Autodesk Fusion 360 part; units mm, degrees
note: some values were not read from the file. Chosen so that the rebuilt part matches the saved one: which bodies a step acts on.
(part 2 of 4)
extrude "Extrude3''''''''''''''" cut sketch "Wedge_Pocket" against normal blind 42.5 from surface at -35 bodies 12 in component "Front_Wedge_L"
sketch "Wedge_HoldDown_Tap" plane through (0, 0, 0) normal (0, 0, 1) x (1, 0, 0) in component "Front_Wedge_L"
  circle A0 centre (-73, 80) radius 1.25
  circle A1 centre (-50, 50) radius 1.25
extrude "Extrude4''''''''''" cut sketch "Wedge_HoldDown_Tap" along normal blind 10 from surface at 5 bodies 12 in component "Front_Wedge_L"
sketch "Wedge_Pocket (2)" plane through (0, 0, 0) normal (1, 0, 0) x (0, 0, -1) in component "Front_Wedge_R"
  line L0 (-7.5, 42.5) -> (-7.5, 85.4279)
  line L1 (-7.5, 85.4279) -> (-74.4675, 42.5)
  line L2 (-74.4675, 42.5) -> (-7.5, 42.5)
extrude "Extrude3'''''''''''''''" cut sketch "Wedge_Pocket (2)" along normal blind 42.5 from surface at 35 bodies 13 in component "Front_Wedge_R"
sketch "Wedge_HoldDown_Tap (2)" plane through (0, 0, 0) normal (0, 0, 1) x (1, 0, 0) in component "Front_Wedge_R"
  circle A0 centre (50, 50) radius 1.25
  circle A1 centre (73, 80) radius 1.25
extrude "Extrude4'''''''''''" cut sketch "Wedge_HoldDown_Tap (2)" along normal blind 10 from surface at 5 bodies 13 in component "Front_Wedge_R"
sketch "Weapon_Pulley_Sketch" plane through (0, 0, 0) normal (1, 0, 0) x (0, 0, -1) in component "Weapon_Pulley"
  circle A0 centre (-38.5, 75) radius 10
extrude "Extrude1'''''''''''''''''''''''''''''" add sketch "Weapon_Pulley_Sketch" along normal blind 6 from surface at 16 separate body makes body 35 in component "Weapon_Pulley"
sketch "Motor_Pulley_Sketch" plane through (0, 0, 0) normal (1, 0, 0) x (0, 0, -1) in component "Motor_Pulley"
  circle A0 centre (-38.5, 25.75) radius 10
extrude "Extrude1''''''''''''''''''''''''''''''" add sketch "Motor_Pulley_Sketch" along normal blind 6 from surface at 16 separate body makes body 36 in component "Motor_Pulley"
sketch "Tension_Slot_-11_16" plane through (0, 0, 0) normal (0, 0, 1) x (1, 0, 0) in component "Base_Plate_Al"
  line L0 (-12.7, 13) -> (-9.3, 13)
  line L1 (-9.3, 13) -> (-9.3, 19)
  line L2 (-9.3, 19) -> (-12.7, 19)
  line L3 (-12.7, 19) -> (-12.7, 13)
extrude "Extrude15'" cut sketch "Tension_Slot_-11_16" along normal blind 6 from surface at 1 bodies 1 in component "Base_Plate_Al"
sketch "Tension_Slot_11_16" plane through (0, 0, 0) normal (0, 0, 1) x (1, 0, 0) in component "Base_Plate_Al"
  line L0 (9.3, 13) -> (12.7, 13)
  line L1 (12.7, 13) -> (12.7, 19)
  line L2 (12.7, 19) -> (9.3, 19)
  line L3 (9.3, 19) -> (9.3, 13)
extrude "Extrude16" cut sketch "Tension_Slot_11_16" along normal blind 6 from surface at 1 bodies 1 in component "Base_Plate_Al"
sketch "Tension_Slot_-11_37" plane through (0, 0, 0) normal (0, 0, 1) x (1, 0, 0) in component "Base_Plate_Al"
  line L0 (-12.7, 34) -> (-9.3, 34)
  line L1 (-9.3, 34) -> (-9.3, 40)
  line L2 (-9.3, 40) -> (-12.7, 40)
  line L3 (-12.7, 40) -> (-12.7, 34)
extrude "Extrude17" cut sketch "Tension_Slot_-11_37" along normal blind 6 from surface at 1 bodies 1 in component "Base_Plate_Al"
sketch "Tension_Slot_11_37" plane through (0, 0, 0) normal (0, 0, 1) x (1, 0, 0) in component "Base_Plate_Al"
  line L0 (9.3, 34) -> (12.7, 34)
  line L1 (12.7, 34) -> (12.7, 40)
  line L2 (12.7, 40) -> (9.3, 40)
  line L3 (9.3, 40) -> (9.3, 34)
extrude "Extrude18" cut sketch "Tension_Slot_11_37" along normal blind 6 from surface at 1 bodies 1 in component "Base_Plate_Al"
sketch "Shaft_Bore" plane through (0, 0, 0) normal (1, 0, 0) x (0, 0, -1) in component "Weapon_Pulley"
  circle A0 centre (-38.5, 75) radius 2
extrude "Extrude2''''''''''''''''''''''''" cut sketch "Shaft_Bore" along normal mid plane 400 bodies 35 in component "Weapon_Pulley"
sketch "Shaft_Bore (2)" plane through (0, 0, 0) normal (1, 0, 0) x (0, 0, -1) in component "Left_Support"
  circle A0 centre (-38.5, 75) radius 2
extrude "Extrude2'''''''''''''''''''''''''" cut sketch "Shaft_Bore (2)" along normal mid plane 400 bodies 15 in component "Left_Support"
sketch "Shaft_Bore (3)" plane through (0, 0, 0) normal (1, 0, 0) x (0, 0, -1) in component "Right_Support"
  circle A0 centre (-38.5, 75) radius 2
extrude "Extrude2''''''''''''''''''''''''''" cut sketch "Shaft_Bore (3)" along normal mid plane 400 bodies 16 in component "Right_Support"
sketch "Shaft_Bore (4)" plane through (0, 0, 0) normal (1, 0, 0) x (0, 0, -1) in component "Motor_Pulley"
  circle A0 centre (-38.5, 25.75) radius 1.585
extrude "Extrude2'''''''''''''''''''''''''''" cut sketch "Shaft_Bore (4)" along normal mid plane 400 bodies 36 in component "Motor_Pulley"
sketch "Wedge_HoldDown_Clear" plane through (0, 0, 0) normal (0, 0, 1) x (1, 0, 0) in component "Front_Wedge_L"
  circle A0 centre (-73, 80) radius 1.7
  circle A1 centre (-50, 50) radius 1.7
extrude "Extrude5'''''''" cut sketch "Wedge_HoldDown_Clear" along normal blind 6 from surface at 4 bodies 12 in component "Front_Wedge_L"
sketch "Wedge_HoldDown_Clear (2)" plane through (0, 0, 0) normal (0, 0, 1) x (1, 0, 0) in component "Front_Wedge_R"
  circle A0 centre (50, 50) radius 1.7
  circle A1 centre (73, 80) radius 1.7
extrude "Extrude5''''''''" cut sketch "Wedge_HoldDown_Clear (2)" along normal blind 6 from surface at 4 bodies 13 in component "Front_Wedge_R"
sketch "ESC_Tekko32_Sketch" plane through (0, 0, 0) normal (0, 0, 1) x (1, 0, 0) in component "ESC_Tekko32"
  line L0 (17.85, 19.35) -> (52.15, 19.35)
  line L1 (52.15, 19.35) -> (52.15, 36.65)
  line L2 (52.15, 36.65) -> (17.85, 36.65)
  line L3 (17.85, 36.65) -> (17.85, 19.35)
extrude "Extrude1'''''''''''''''''''''''''''''''" add sketch "ESC_Tekko32_Sketch" along normal blind 4.5 from surface at 7 separate body makes body 37 in component "ESC_Tekko32"
sketch "Holder_ESC_Tekko32_Sketch" plane through (0, 0, 0) normal (0, 0, 1) x (1, 0, 0) in component "Holder_ESC_Tekko32"
  line L0 (16.05, 17.55) -> (53.95, 17.55)
  line L1 (53.95, 17.55) -> (53.95, 38.45)
  line L2 (53.95, 38.45) -> (16.05, 38.45)
  line L3 (16.05, 38.45) -> (16.05, 17.55)
extrude "Extrude1''''''''''''''''''''''''''''''''" add sketch "Holder_ESC_Tekko32_Sketch" along normal blind 5.5 from surface at 5 separate body makes body 38 in component "Holder_ESC_Tekko32"
sketch "Holder_ESC_Tekko32_Pocket" plane through (0, 0, 0) normal (0, 0, 1) x (1, 0, 0) in component "Holder_ESC_Tekko32"
  line L0 (17.65, 19.15) -> (52.35, 19.15)
  line L1 (52.35, 19.15) -> (52.35, 36.85)
  line L2 (52.35, 36.85) -> (17.65, 36.85)
  line L3 (17.65, 36.85) -> (17.65, 19.15)
extrude "Extrude2''''''''''''''''''''''''''''" cut sketch "Holder_ESC_Tekko32_Pocket" along normal blind 60 from surface at 7 bodies 38 in component "Holder_ESC_Tekko32"
sketch "Holder_ESC_Tekko32_TieGroove" plane through (0, 0, 0) normal (0, 0, 1) x (1, 0, 0) in component "Holder_ESC_Tekko32"
  line L0 (33, 16.55) -> (37, 16.55)
  line L1 (37, 16.55) -> (37, 39.45)
  line L2 (37, 39.45) -> (33, 39.45)
  line L3 (33, 39.45) -> (33, 16.55)
extrude "Extrude3''''''''''''''''" cut sketch "Holder_ESC_Tekko32_TieGroove" along normal blind 2.2 from surface at 4 bodies 38 in component "Holder_ESC_Tekko32"
sketch "Holder_ESC_Tekko32_FloorHoles" plane through (0, 0, 0) normal (0, 0, 1) x (1, 0, 0) in component "Holder_ESC_Tekko32"
  circle A0 centre (21.85, 28) radius 1.7
  circle A1 centre (48.15, 28) radius 1.7
extrude "Extrude4''''''''''''" cut sketch "Holder_ESC_Tekko32_FloorHoles" along normal blind 4 from surface at 4 bodies 38 in component "Holder_ESC_Tekko32"
sketch "Holder_ESC_Tekko32_PlateHoles" plane through (0, 0, 0) normal (0, 0, 1) x (1, 0, 0) in component "Base_Plate_Al"
  circle A0 centre (21.85, 28) radius 1.25
  circle A1 centre (48.15, 28) radius 1.25
extrude "Extrude23" cut sketch "Holder_ESC_Tekko32_PlateHoles" along normal blind 6 from surface at 1 bodies 1 in component "Base_Plate_Al"
sketch "Rx_ER6_Sketch" plane through (0, 0, 0) normal (0, 0, 1) x (1, 0, 0) in component "Rx_ER6"
  line L0 (-64.5, -84.5) -> (-39.5, -84.5)
  line L1 (-39.5, -84.5) -> (-39.5, -41.5)
  line L2 (-39.5, -41.5) -> (-64.5, -41.5)
  line L3 (-64.5, -41.5) -> (-64.5, -84.5)
extrude "Extrude1'''''''''''''''''''''''''''''''''" add sketch "Rx_ER6_Sketch" along normal blind 15 from surface at 7 separate body makes body 39 in component "Rx_ER6"
sketch "Holder_Rx_ER6_Sketch" plane through (0, 0, 0) normal (0, 0, 1) x (1, 0, 0) in component "Holder_Rx_ER6"
  line L0 (-66.3, -86.3) -> (-37.7, -86.3)
  line L1 (-37.7, -86.3) -> (-37.7, -39.7)
  line L2 (-37.7, -39.7) -> (-66.3, -39.7)
  line L3 (-66.3, -39.7) -> (-66.3, -86.3)
extrude "Extrude1''''''''''''''''''''''''''''''''''" add sketch "Holder_Rx_ER6_Sketch" along normal blind 16 from surface at 5 separate body makes body 40 in component "Holder_Rx_ER6"
sketch "Holder_Rx_ER6_Pocket" plane through (0, 0, 0) normal (0, 0, 1) x (1, 0, 0) in component "Holder_Rx_ER6"
  line L0 (-64.7, -84.7) -> (-39.3, -84.7)
  line L1 (-39.3, -84.7) -> (-39.3, -41.3)
  line L2 (-39.3, -41.3) -> (-64.7, -41.3)
  line L3 (-64.7, -41.3) -> (-64.7, -84.7)
extrude "Extrude2'''''''''''''''''''''''''''''" cut sketch "Holder_Rx_ER6_Pocket" along normal blind 60 from surface at 7 bodies 40 in component "Holder_Rx_ER6"
sketch "Holder_Rx_ER6_TieGroove" plane through (0, 0, 0) normal (0, 0, 1) x (1, 0, 0) in component "Holder_Rx_ER6"
  line L0 (-67.3, -65) -> (-36.7, -65)
  line L1 (-36.7, -65) -> (-36.7, -61)
  line L2 (-36.7, -61) -> (-67.3, -61)
  line L3 (-67.3, -61) -> (-67.3, -65)
extrude "Extrude3'''''''''''''''''" cut sketch "Holder_Rx_ER6_TieGroove" along normal blind 2.2 from surface at 4 bodies 40 in component "Holder_Rx_ER6"
sketch "Holder_Rx_ER6_FloorHoles" plane through (0, 0, 0) normal (0, 0, 1) x (1, 0, 0) in component "Holder_Rx_ER6"
  circle A0 centre (-52, -80.5) radius 1.7
  circle A1 centre (-52, -45.5) radius 1.7
extrude "Extrude4'''''''''''''" cut sketch "Holder_Rx_ER6_FloorHoles" along normal blind 4 from surface at 4 bodies 40 in component "Holder_Rx_ER6"
sketch "Holder_Rx_ER6_PlateHoles" plane through (0, 0, 0) normal (0, 0, 1) x (1, 0, 0) in component "Base_Plate_Al"
  circle A0 centre (-52, -80.5) radius 1.25
  circle A1 centre (-52, -45.5) radius 1.25
extrude "Extrude24" cut sketch "Holder_Rx_ER6_PlateHoles" along normal blind 6 from surface at 1 bodies 1 in component "Base_Plate_Al"
sketch "UBEC_5A_Sketch" plane through (0, 0, 0) normal (0, 0, 1) x (1, 0, 0) in component "UBEC_5A"
  line L0 (57.5, -76) -> (74.5, -76)
  line L1 (74.5, -76) -> (74.5, -26)
  line L2 (74.5, -26) -> (57.5, -26)
  line L3 (57.5, -26) -> (57.5, -76)
extrude "Extrude1'''''''''''''''''''''''''''''''''''" add sketch "UBEC_5A_Sketch" along normal blind 10 from surface at 7 separate body makes body 41 in component "UBEC_5A"
sketch "Holder_UBEC_5A_Sketch" plane through (0, 0, 0) normal (0, 0, 1) x (1, 0, 0) in component "Holder_UBEC_5A"
  line L0 (55.7, -77.8) -> (76.3, -77.8)
  line L1 (76.3, -77.8) -> (76.3, -24.2)
  line L2 (76.3, -24.2) -> (55.7, -24.2)
  line L3 (55.7, -24.2) -> (55.7, -77.8)
extrude "Extrude1''''''''''''''''''''''''''''''''''''" add sketch "Holder_UBEC_5A_Sketch" along normal blind 11 from surface at 5 separate body makes body 42 in component "Holder_UBEC_5A"
sketch "Holder_UBEC_5A_Pocket" plane through (0, 0, 0) normal (0, 0, 1) x (1, 0, 0) in component "Holder_UBEC_5A"
  line L0 (57.3, -76.2) -> (74.7, -76.2)
  line L1 (74.7, -76.2) -> (74.7, -25.8)
  line L2 (74.7, -25.8) -> (57.3, -25.8)
  line L3 (57.3, -25.8) -> (57.3, -76.2)
extrude "Extrude2''''''''''''''''''''''''''''''" cut sketch "Holder_UBEC_5A_Pocket" along normal blind 60 from surface at 7 bodies 42 in component "Holder_UBEC_5A"
sketch "Holder_UBEC_5A_TieGroove" plane through (0, 0, 0) normal (0, 0, 1) x (1, 0, 0) in component "Holder_UBEC_5A"
  line L0 (54.7, -53) -> (77.3, -53)
  line L1 (77.3, -53) -> (77.3, -49)
  line L2 (77.3, -49) -> (54.7, -49)
  line L3 (54.7, -49) -> (54.7, -53)
extrude "Extrude3''''''''''''''''''" cut sketch "Holder_UBEC_5A_TieGroove" along normal blind 2.2 from surface at 4 bodies 42 in component "Holder_UBEC_5A"
sketch "Holder_UBEC_5A_FloorHoles" plane through (0, 0, 0) normal (0, 0, 1) x (1, 0, 0) in component "Holder_UBEC_5A"
  circle A0 centre (66, -72) radius 1.7
  circle A1 centre (66, -30) radius 1.7
extrude "Extrude4''''''''''''''" cut sketch "Holder_UBEC_5A_FloorHoles" along normal blind 4 from surface at 4 bodies 42 in component "Holder_UBEC_5A"
sketch "Holder_UBEC_5A_PlateHoles" plane through (0, 0, 0) normal (0, 0, 1) x (1, 0, 0) in component "Base_Plate_Al"
  circle A0 centre (66, -72) radius 1.25
  circle A1 centre (66, -30) radius 1.25
extrude "Extrude25" cut sketch "Holder_UBEC_5A_PlateHoles" along normal blind 6 from surface at 1 bodies 1 in component "Base_Plate_Al"
sketch "DRV8874_A_Sketch" plane through (0, 0, 0) normal (0, 0, 1) x (1, 0, 0) in component "DRV8874_A"
  line L0 (-34.9, -81.6) -> (-17.1, -81.6)
  line L1 (-17.1, -81.6) -> (-17.1, -66.4)
  line L2 (-17.1, -66.4) -> (-34.9, -66.4)
  line L3 (-34.9, -66.4) -> (-34.9, -81.6)
extrude "Extrude1'''''''''''''''''''''''''''''''''''''" add sketch "DRV8874_A_Sketch" along normal blind 3 from surface at 7 separate body makes body 43 in component "DRV8874_A"
sketch "Holder_DRV8874_A_Sketch" plane through (0, 0, 0) normal (0, 0, 1) x (1, 0, 0) in component "Holder_DRV8874_A"
  line L0 (-36.7, -83.4) -> (-15.3, -83.4)
  line L1 (-15.3, -83.4) -> (-15.3, -64.6)
  line L2 (-15.3, -64.6) -> (-36.7, -64.6)
  line L3 (-36.7, -64.6) -> (-36.7, -83.4)
extrude "Extrude1''''''''''''''''''''''''''''''''''''''" add sketch "Holder_DRV8874_A_Sketch" along normal blind 4 from surface at 5 separate body makes body 44 in component "Holder_DRV8874_A"
sketch "Holder_DRV8874_A_Pocket" plane through (0, 0, 0) normal (0, 0, 1) x (1, 0, 0) in component "Holder_DRV8874_A"
  line L0 (-35.1, -81.8) -> (-16.9, -81.8)
  line L1 (-16.9, -81.8) -> (-16.9, -66.2)
  line L2 (-16.9, -66.2) -> (-35.1, -66.2)
  line L3 (-35.1, -66.2) -> (-35.1, -81.8)
extrude "Extrude2'''''''''''''''''''''''''''''''" cut sketch "Holder_DRV8874_A_Pocket" along normal blind 60 from surface at 7 bodies 44 in component "Holder_DRV8874_A"
sketch "Holder_DRV8874_A_TieGroove" plane through (0, 0, 0) normal (0, 0, 1) x (1, 0, 0) in component "Holder_DRV8874_A"
  line L0 (-28, -84.4) -> (-24, -84.4)
  line L1 (-24, -84.4) -> (-24, -63.6)
  line L2 (-24, -63.6) -> (-28, -63.6)
  line L3 (-28, -63.6) -> (-28, -84.4)
extrude "Extrude3'''''''''''''''''''" cut sketch "Holder_DRV8874_A_TieGroove" along normal blind 2.2 from surface at 4 bodies 44 in component "Holder_DRV8874_A"
sketch "Holder_DRV8874_A_FloorHoles" plane through (0, 0, 0) normal (0, 0, 1) x (1, 0, 0) in component "Holder_DRV8874_A"
  circle A0 centre (-31, -74) radius 1.7
  circle A1 centre (-21, -74) radius 1.7
extrude "Extrude4'''''''''''''''" cut sketch "Holder_DRV8874_A_FloorHoles" along normal blind 4 from surface at 4 bodies 44 in component "Holder_DRV8874_A"
sketch "Holder_DRV8874_A_PlateHoles" plane through (0, 0, 0) normal (0, 0, 1) x (1, 0, 0) in component "Base_Plate_Al"
  circle A0 centre (-31, -74) radius 1.25
  circle A1 centre (-21, -74) radius 1.25
extrude "Extrude26" cut sketch "Holder_DRV8874_A_PlateHoles" along normal blind 6 from surface at 1 bodies 1 in component "Base_Plate_Al"
sketch "DRV8874_B_Sketch" plane through (0, 0, 0) normal (0, 0, 1) x (1, 0, 0) in component "DRV8874_B"
  line L0 (-11.6, -83.9) -> (3.6, -83.9)
  line L1 (3.6, -83.9) -> (3.6, -66.1)
  line L2 (3.6, -66.1) -> (-11.6, -66.1)
  line L3 (-11.6, -66.1) -> (-11.6, -83.9)
extrude "Extrude1'''''''''''''''''''''''''''''''''''''''" add sketch "DRV8874_B_Sketch" along normal blind 3 from surface at 7 separate body makes body 45 in component "DRV8874_B"
sketch "Holder_DRV8874_B_Sketch" plane through (0, 0, 0) normal (0, 0, 1) x (1, 0, 0) in component "Holder_DRV8874_B"
  line L0 (-13.4, -85.7) -> (5.4, -85.7)
  line L1 (5.4, -85.7) -> (5.4, -64.3)
  line L2 (5.4, -64.3) -> (-13.4, -64.3)
  line L3 (-13.4, -64.3) -> (-13.4, -85.7)
extrude "Extrude1''''''''''''''''''''''''''''''''''''''''" add sketch "Holder_DRV8874_B_Sketch" along normal blind 4 from surface at 5 separate body makes body 46 in component "Holder_DRV8874_B"
sketch "Holder_DRV8874_B_Pocket" plane through (0, 0, 0) normal (0, 0, 1) x (1, 0, 0) in component "Holder_DRV8874_B"
  line L0 (-11.8, -84.1) -> (3.8, -84.1)
  line L1 (3.8, -84.1) -> (3.8, -65.9)
  line L2 (3.8, -65.9) -> (-11.8, -65.9)
  line L3 (-11.8, -65.9) -> (-11.8, -84.1)
extrude "Extrude2''''''''''''''''''''''''''''''''" cut sketch "Holder_DRV8874_B_Pocket" along normal blind 60 from surface at 7 bodies 46 in component "Holder_DRV8874_B"
sketch "Holder_DRV8874_B_TieGroove" plane through (0, 0, 0) normal (0, 0, 1) x (1, 0, 0) in component "Holder_DRV8874_B"
  line L0 (-14.4, -77) -> (6.4, -77)
  line L1 (6.4, -77) -> (6.4, -73)
  line L2 (6.4, -73) -> (-14.4, -73)
  line L3 (-14.4, -73) -> (-14.4, -77)
extrude "Extrude3''''''''''''''''''''" cut sketch "Holder_DRV8874_B_TieGroove" along normal blind 2.2 from surface at 4 bodies 46 in component "Holder_DRV8874_B"
sketch "Holder_DRV8874_B_FloorHoles" plane through (0, 0, 0) normal (0, 0, 1) x (1, 0, 0) in component "Holder_DRV8874_B"
  circle A0 centre (-4, -80) radius 1.7
  circle A1 centre (-4, -70) radius 1.7
extrude "Extrude4''''''''''''''''" cut sketch "Holder_DRV8874_B_FloorHoles" along normal blind 4 from surface at 4 bodies 46 in component "Holder_DRV8874_B"
sketch "Holder_DRV8874_B_PlateHoles" plane through (0, 0, 0) normal (0, 0, 1) x (1, 0, 0) in component "Base_Plate_Al"
  circle A0 centre (-4, -80) radius 1.25
  circle A1 centre (-4, -70) radius 1.25
extrude "Extrude27" cut sketch "Holder_DRV8874_B_PlateHoles" along normal blind 6 from surface at 1 bodies 1 in component "Base_Plate_Al"
sketch "ESP32_DevKit_Sketch" plane through (0, 0, 0) normal (0, 0, 1) x (1, 0, 0) in component "ESP32_DevKit"
  line L0 (-25.75, -52.15) -> (25.75, -52.15)
  line L1 (25.75, -52.15) -> (25.75, -23.85)
  line L2 (25.75, -23.85) -> (-25.75, -23.85)
  line L3 (-25.75, -23.85) -> (-25.75, -52.15)
extrude "Extrude1'''''''''''''''''''''''''''''''''''''''''" add sketch "ESP32_DevKit_Sketch" along normal blind 1.6 from surface at 25 separate body makes body 47 in component "ESP32_DevKit"
sketch "ESP32_Holes" plane through (0, 0, 0) normal (0, 0, 1) x (1, 0, 0) in component "ESP32_DevKit"
  circle A0 centre (-23.6, -49.7) radius 1.3
  circle A1 centre (-23.6, -26.3) radius 1.3
  circle A2 centre (23.6, -49.7) radius 1.3
  circle A3 centre (23.6, -26.3) radius 1.3
extrude "Extrude2'''''''''''''''''''''''''''''''''" cut sketch "ESP32_Holes" along normal blind 3.6 from surface at 24 bodies 47 in component "ESP32_DevKit"
sketch "ESP32_Module_Sketch" plane through (0, 0, 0) normal (0, 0, 1) x (1, 0, 0) in component "ESP32_DevKit"
  line L0 (-25.75, -47) -> (-0.25, -47)
  line L1 (-0.25, -47) -> (-0.25, -29)
  line L2 (-0.25, -29) -> (-25.75, -29)
  line L3 (-25.75, -29) -> (-25.75, -47)
extrude "Extrude3'''''''''''''''''''''" add sketch "ESP32_Module_Sketch" along normal blind 3.1 from surface at 26.6 separate body makes body 48 in component "ESP32_DevKit"
sketch "ESP32_Dupont_Keepout_A_Sketch" plane through (0, 0, 0) normal (0, 0, 1) x (1, 0, 0) in component "ESP32_DevKit"
  line L0 (-20.72, -51.97) -> (14.88, -51.97)
  line L1 (14.88, -51.97) -> (14.88, -49.43)
  line L2 (14.88, -49.43) -> (-20.72, -49.43)
  line L3 (-20.72, -49.43) -> (-20.72, -51.97)
extrude "Extrude4'''''''''''''''''" add sketch "ESP32_Dupont_Keepout_A_Sketch" along normal blind 16.5 from surface at 8.5 separate body makes body 49 in component "ESP32_DevKit"
sketch "ESP32_Dupont_Keepout_B_Sketch" plane through (0, 0, 0) normal (0, 0, 1) x (1, 0, 0) in component "ESP32_DevKit"
  line L0 (-20.72, -26.57) -> (14.88, -26.57)
  line L1 (14.88, -26.57) -> (14.88, -24.03)
  line L2 (14.88, -24.03) -> (-20.72, -24.03)
  line L3 (-20.72, -24.03) -> (-20.72, -26.57)
extrude "Extrude5'''''''''" add sketch "ESP32_Dupont_Keepout_B_Sketch" along normal blind 16.5 from surface at 8.5 separate body makes body 50 in component "ESP32_DevKit"
sketch "Holder_ESP32_Sketch" plane through (0, 0, 0) normal (0, 0, 1) x (1, 0, 0) in component "Holder_ESP32"
  line L0 (-27.75, -54.15) -> (27.75, -54.15)
  line L1 (27.75, -54.15) -> (27.75, -21.85)
  line L2 (27.75, -21.85) -> (-27.75, -21.85)
  line L3 (-27.75, -21.85) -> (-27.75, -54.15)
extrude "Extrude1''''''''''''''''''''''''''''''''''''''''''" add sketch "Holder_ESP32_Sketch" along normal blind 2 from surface at 5 separate body makes body 51 in component "Holder_ESP32"
sketch "Holder_ESP32_Posts" plane through (0, 0, 0) normal (0, 0, 1) x (1, 0, 0) in component "Holder_ESP32"
  circle A0 centre (-23.6, -49.7) radius 2.25
  circle A1 centre (-23.6, -26.3) radius 2.25
  circle A2 centre (23.6, -49.7) radius 2.25
  circle A3 centre (23.6, -26.3) radius 2.25
extrude "Extrude2''''''''''''''''''''''''''''''''''" add sketch "Holder_ESP32_Posts" along normal blind 18 from surface at 7 bodies 51 in component "Holder_ESP32"
sketch "Holder_ESP32_Window" plane through (0, 0, 0) normal (0, 0, 1) x (1, 0, 0) in component "Holder_ESP32"
  line L0 (-9, -47.15) -> (9, -47.15)
  line L1 (9, -47.15) -> (9, -28.85)
  line L2 (9, -28.85) -> (-9, -28.85)
  line L3 (-9, -28.85) -> (-9, -47.15)
extrude "Extrude3''''''''''''''''''''''" cut sketch "Holder_ESP32_Window" along normal blind 4 from surface at 4 bodies 51 in component "Holder_ESP32"
sketch "Holder_ESP32_PostPilots" plane through (0, 0, 0) normal (0, 0, 1) x (1, 0, 0) in component "Holder_ESP32"
  circle A0 centre (-23.6, -49.7) radius 0.8
  circle A1 centre (-23.6, -26.3) radius 0.8
  circle A2 centre (23.6, -49.7) radius 0.8
  circle A3 centre (23.6, -26.3) radius 0.8
extrude "Extrude4''''''''''''''''''" cut sketch "Holder_ESP32_PostPilots" against normal blind 8 from surface at 25 bodies 51 in component "Holder_ESP32"
sketch "Holder_ESP32_Screws" plane through (0, 0, 0) normal (0, 0, 1) x (1, 0, 0) in component "Holder_ESP32"
  circle A0 centre (-15, -38) radius 1.7
  circle A1 centre (15, -38) radius 1.7
extrude "Extrude5''''''''''" cut sketch "Holder_ESP32_Screws" along normal blind 4 from surface at 4 bodies 51 in component "Holder_ESP32"
sketch "Holder_ESP32_PlateHoles" plane through (0, 0, 0) normal (0, 0, 1) x (1, 0, 0) in component "Base_Plate_Al"
  circle A0 centre (-15, -38) radius 1.25
  circle A1 centre (15, -38) radius 1.25
extrude "Extrude28" cut sketch "Holder_ESP32_PlateHoles" along normal blind 6 from surface at 1 bodies 1 in component "Base_Plate_Al"
sketch "DXF_Base_Plate_Al" plane through (0, 0, 3) normal (0, 0, -1) x (-1, 0, 0) in component "Base_Plate_Al"
  circle A0 centre (4, -80) radius 1.25
  circle A1 centre (4, -70) radius 1.25
  circle A2 centre (-66, -72) radius 1.25
  circle A3 centre (-66, -30) radius 1.25
  circle A4 centre (-21.85, 28) radius 1.25
  circle A5 centre (-48.15, 28) radius 1.25
  line L0 (12.7, 40) -> (12.7, 34)
  line L1 (12.7, 34) -> (9.3, 34)
  line L2 (9.3, 34) -> (9.3, 40)
  line L3 (9.3, 40) -> (12.7, 40)
  line L4 (12.7, 19) -> (12.7, 13)
  line L5 (12.7, 13) -> (9.3, 13)
  line L6 (9.3, 13) -> (9.3, 19)
  line L7 (9.3, 19) -> (12.7, 19)
  circle A6 centre (34, -46) radius 1.45
  circle A7 centre (-34, -30) radius 1.45
  circle A8 centre (34, -30) radius 1.45
  circle A9 centre (-34, -46) radius 1.45
  circle A10 centre (38.7, -14) radius 1.7
  circle A11 centre (51, 14) radius 1.7
  circle A12 centre (51, -14) radius 1.7
  circle A13 centre (38.7, 14) radius 1.7
  circle A14 centre (-73, 80) radius 1.7
  circle A15 centre (-50, 50) radius 1.7
  circle A16 centre (73, 80) radius 1.7
  circle A17 centre (50, 50) radius 1.7
  circle A18 centre (75, 35) radius 1.7
  circle A19 centre (-75, -85) radius 1.7
  circle A20 centre (75, -85) radius 1.7
  circle A21 centre (-75, 35) radius 1.7
  line L8 (-80, 24) -> (-58, 24)
  line L9 (-58, 24) -> (-58, -24)
  line L10 (-58, -24) -> (-80, -24)
  line L11 (-80, -24) -> (-80, -90)
  line L12 (-80, -90) -> (80, -90)
  line L13 (80, -90) -> (80, -24)
  line L14 (80, -24) -> (58, -24)
  line L15 (58, -24) -> (58, 24)
  line L16 (58, 24) -> (80, 24)
  line L17 (80, 24) -> (80, 90)
  line L18 (80, 90) -> (-80, 90)
  line L19 (-80, 90) -> (-80, 24)
  circle A22 centre (-51, 14) radius 1.7
  circle A23 centre (-38.7, -14) radius 1.7
  circle A24 centre (-38.7, 14) radius 1.7
  circle A25 centre (-51, -14) radius 1.7
  circle A26 centre (-51.5, -70) radius 1.45
  circle A27 centre (-32.5, -70) radius 1.45
  line L20 (-9.3, 19) -> (-9.3, 13)
  line L21 (-9.3, 13) -> (-12.7, 13)
  line L22 (-12.7, 13) -> (-12.7, 19)
  line L23 (-12.7, 19) -> (-9.3, 19)
  line L24 (-9.3, 40) -> (-9.3, 34)
  line L25 (-9.3, 34) -> (-12.7, 34)
  line L26 (-12.7, 34) -> (-12.7, 40)
  line L27 (-12.7, 40) -> (-9.3, 40)
  circle A28 centre (52, -45.5) radius 1.25
  circle A29 centre (52, -80.5) radius 1.25
  circle A30 centre (21, -74) radius 1.25
  circle A31 centre (31, -74) radius 1.25
  circle A32 centre (-15, -38) radius 1.25
  circle A33 centre (15, -38) radius 1.25
sketch "DXF_Left_Side_Plate_Al" plane through (-78, 0, 0) normal (1, 0, 0) x (0, 0, -1) in component "Left_Side_Plate_Al"
  circle A0 centre (-44, -85) radius 1.7
  circle A1 centre (-44, 35) radius 1.7
  line L0 (-5, -26) -> (-47, -26)
  line L1 (-47, -26) -> (-47, 26)
  line L2 (-47, 26) -> (-5, 26)
  line L3 (-5, 26) -> (-5, 40)
  line L4 (-5, 40) -> (-83, 40)
  line L5 (-83, 40) -> (-83, -90)
  line L6 (-83, -90) -> (-5, -90)
  line L7 (-5, -90) -> (-5, -26)
sketch "DXF_Right_Side_Plate_Al" plane through (78, 0, 0) normal (-1, 0, 0) x (0, 0, 1) in component "Right_Side_Plate_Al"
  circle A0 centre (44, -85) radius 1.7
  circle A1 centre (44, 35) radius 1.7
  line L0 (5, 26) -> (47, 26)
  line L1 (47, 26) -> (47, -26)
  line L2 (47, -26) -> (5, -26)
  line L3 (5, -26) -> (5, -90)
  line L4 (5, -90) -> (83, -90)
  line L5 (83, -90) -> (83, 40)
  line L6 (83, 40) -> (5, 40)
  line L7 (5, 40) -> (5, 26)
sketch "DXF_Front_Wedge_L" plane through (-80, 0, 0) normal (-1, 0, 0) x (0, 0, 1) in component "Front_Wedge_L"
  line L0 (5, 40) -> (83, 40)
  line L1 (83, 40) -> (5, 90)
  line L2 (5, 90) -> (5, 40)
sketch "DXF_Front_Wedge_R" plane through (80, 0, 0) normal (1, 0, 0) x (0, 0, -1) in component "Front_Wedge_R"
  line L0 (-83, 40) -> (-5, 40)
  line L1 (-5, 40) -> (-5, 90)
  line L2 (-5, 90) -> (-83, 40)
sketch "FingerTech_Switch_Adapter_Outline" plane through (0, 0, 0) normal (0, 0, 1) x (1, 0, 0) in component "FingerTech_Switch_Adapter"
  line L0 (28, -79) -> (56, -79)
  line L1 (56, -79) -> (56, -61)
  line L2 (56, -61) -> (28, -61)
  line L3 (28, -61) -> (28, -79)
extrude "Extrude1'''''''''''''''''''''''''''''''''''''''''''" add sketch "FingerTech_Switch_Adapter_Outline" along normal blind 4 from surface at 45 separate body makes body 52 in component "FingerTech_Switch_Adapter"
sketch "Adapter_Post_Clearance_M3" plane through (0, 0, 0) normal (0, 0, 1) x (1, 0, 0) in component "FingerTech_Switch_Adapter"
  circle A0 centre (32.5, -70) radius 1.7
  circle A1 centre (51.5, -70) radius 1.7
extrude "Extrude2'''''''''''''''''''''''''''''''''''" cut sketch "Adapter_Post_Clearance_M3" along normal blind 6 from surface at 44 bodies 52 in component "FingerTech_Switch_Adapter"
sketch "Adapter_Switch_Clearance_M2" plane through (0, 0, 0) normal (0, 0, 1) x (1, 0, 0) in component "FingerTech_Switch_Adapter"
  circle A0 centre (38.19, -70) radius 1.1
  circle A1 centre (45.81, -70) radius 1.1
extrude "Extrude3'''''''''''''''''''''''" cut sketch "Adapter_Switch_Clearance_M2" along normal blind 6 from surface at 44 bodies 52 in component "FingerTech_Switch_Adapter"
sketch "FingerTech_Mini_Switch_Envelope_Outline" plane through (0, 0, 0) normal (0, 0, 1) x (1, 0, 0) in component "FingerTech_Mini_Switch_Envelope"
  line L0 (35.65, -76.35) -> (48.35, -76.35)
  line L1 (48.35, -76.35) -> (48.35, -63.65)
  line L2 (48.35, -63.65) -> (35.65, -63.65)
  line L3 (35.65, -63.65) -> (35.65, -76.35)
extrude "Extrude1''''''''''''''''''''''''''''''''''''''''''''" add sketch "FingerTech_Mini_Switch_Envelope_Outline" along normal blind 6.35 from surface at 49 separate body makes body 53 in component "FingerTech_Mini_Switch_Envelope"
sketch "FingerTech_Mount_Holes_M2" plane through (0, 0, 0) normal (0, 0, 1) x (1, 0, 0) in component "FingerTech_Mini_Switch_Envelope"
  circle A0 centre (38.19, -70) radius 1
  circle A1 centre (45.81, -70) radius 1
extrude "Extrude2''''''''''''''''''''''''''''''''''''" cut sketch "FingerTech_Mount_Holes_M2" along normal blind 9 from surface at 48 bodies 53 in component "FingerTech_Mini_Switch_Envelope"
sketch "FingerTech_Access_Patch" plane through (0, 0, 0) normal (0, 0, 1) x (1, 0, 0) in component "Top_Cover"
  line L0 (31, -79) -> (53, -79)
  line L1 (53, -79) -> (53, -61)
  line L2 (53, -61) -> (31, -61)
  line L3 (31, -61) -> (31, -79)
extrude "Extrude7''''" add sketch "FingerTech_Access_Patch" along normal blind 2 from surface at 83 bodies 6 in component "Top_Cover"
sketch "FingerTech_Hex_Access_6mm" plane through (0, 0, 0) normal (0, 0, 1) x (1, 0, 0) in component "Top_Cover"
  circle A0 centre (42, -70) radius 3
extrude "Extrude8''" cut sketch "FingerTech_Hex_Access_6mm" along normal blind 4 from surface at 82 bodies 6 in component "Top_Cover"
sketch "Original_Vertical_Bar_6x65" plane through (0, 0, 0) normal (0, 0, 1) x (1, 0, 0) in component "Spinner_Bar"
  line L0 (-3, 42.5) -> (3, 42.5)
  line L1 (3, 42.5) -> (3, 107.5)
  line L2 (3, 107.5) -> (-3, 107.5)
  line L3 (-3, 107.5) -> (-3, 42.5)
extrude "Extrude1'''''''''''''''''''''''''''''''''''''''''''''" add sketch "Original_Vertical_Bar_6x65" along normal blind 20 from surface at 28.5 separate body makes body 54 in component "Spinner_Bar"
sketch "Existing_Shaft_4mm_Bore_Provisional" plane through (0, 0, 0) normal (1, 0, 0) x (0, 0, -1) in component "Spinner_Bar"
  circle A0 centre (-38.5, 75) radius 2
extrude "Extrude2'''''''''''''''''''''''''''''''''''''" cut sketch "Existing_Shaft_4mm_Bore_Provisional" along normal mid plane 10 bodies 54 in component "Spinner_Bar"
sketch "Original_Bar_Rotation_Radius_32p5" plane through (0, 0, 0) normal (1, 0, 0) x (0, 0, -1) in component "Spinner_Sweep_Envelope"
  circle A0 centre (-38.5, 75) radius 32.5
extrude "Extrude1''''''''''''''''''''''''''''''''''''''''''''''" add sketch "Original_Bar_Rotation_Radius_32p5" along normal blind 6 from surface at -3 separate body makes body 55 in component "Spinner_Sweep_Envelope"
sketch "Lifter_Spatula_62mm_Side_Profile" plane through (0, 0, 0) normal (1, 0, 0) x (0, 0, -1) in component "Lifter_Spatula_62mm"
  line L0 (-27, 70) -> (-5.8, 112)
  line L1 (-5.8, 112) -> (-8.5, 112)
  line L2 (-8.5, 112) -> (-30, 72)
  line L3 (-30, 72) -> (-27, 70)
extrude "Extrude1'''''''''''''''''''''''''''''''''''''''''''''''" add sketch "Lifter_Spatula_62mm_Side_Profile" along normal blind 62 from surface at -31 separate body makes body 56 in component "Lifter_Spatula_62mm"
sketch "Lifter_Hinge_Boss_Outline" plane through (0, 0, 0) normal (0, 0, 1) x (1, 0, 0) in component "Lifter_Hinge_Boss"
  line L0 (-30, 64) -> (30, 64)
  line L1 (30, 64) -> (30, 74)
  line L2 (30, 74) -> (-30, 74)
  line L3 (-30, 74) -> (-30, 64)
extrude "Extrude1''''''''''''''''''''''''''''''''''''''''''''''''" add sketch "Lifter_Hinge_Boss_Outline" along normal blind 9 from surface at 27 separate body makes body 57 in component "Lifter_Hinge_Boss"
sketch "Hinge_Clearance_Bore_6p4mm" plane through (0, 0, 0) normal (1, 0, 0) x (0, 0, -1) in component "Lifter_Hinge_Boss"
  circle A0 centre (-31.5, 68) radius 3.2
extrude "Extrude2''''''''''''''''''''''''''''''''''''''" cut sketch "Hinge_Clearance_Bore_6p4mm" along normal mid plane 100 bodies 57 in component "Lifter_Hinge_Boss"
sketch "Lifter_Pivot_Support_L_Outline" plane through (0, 0, 0) normal (0, 0, 1) x (1, 0, 0) in component "Lifter_Pivot_Support_L"
  line L0 (-35, 61) -> (-32, 61)
  line L1 (-32, 61) -> (-32, 76)
  line L2 (-32, 76) -> (-35, 76)
  line L3 (-35, 76) -> (-35, 61)
extrude "Extrude1'''''''''''''''''''''''''''''''''''''''''''''''''" add sketch "Lifter_Pivot_Support_L_Outline" along normal blind 17 from surface at 24 separate body makes body 58 in component "Lifter_Pivot_Support_L"
sketch "Lifter_Pivot_Support_R_Outline" plane through (0, 0, 0) normal (0, 0, 1) x (1, 0, 0) in component "Lifter_Pivot_Support_R"
  line L0 (32, 61) -> (35, 61)
  line L1 (35, 61) -> (35, 76)
  line L2 (35, 76) -> (32, 76)
  line L3 (32, 76) -> (32, 61)
extrude "Extrude1''''''''''''''''''''''''''''''''''''''''''''''''''" add sketch "Lifter_Pivot_Support_R_Outline" along normal blind 17 from surface at 24 separate body makes body 59 in component "Lifter_Pivot_Support_R"
sketch "Left_Pivot_Bore_6p4mm" plane through (0, 0, 0) normal (1, 0, 0) x (0, 0, -1) in component "Lifter_Pivot_Support_L"
  circle A0 centre (-31.5, 68) radius 3.2
extrude "Extrude2'''''''''''''''''''''''''''''''''''''''" cut sketch "Left_Pivot_Bore_6p4mm" along normal mid plane 100 bodies 58 in component "Lifter_Pivot_Support_L"
sketch "Right_Pivot_Bore_6p4mm" plane through (0, 0, 0) normal (1, 0, 0) x (0, 0, -1) in component "Lifter_Pivot_Support_R"
  circle A0 centre (-31.5, 68) radius 3.2
extrude "Extrude2''''''''''''''''''''''''''''''''''''''''" cut sketch "Right_Pivot_Bore_6p4mm" along normal mid plane 100 bodies 59 in component "Lifter_Pivot_Support_R"
sketch "Lifter_Pivot_Pin_6mm_Section" plane through (0, 0, 0) normal (1, 0, 0) x (0, 0, -1) in component "Lifter_Pivot_Pin_6mm"
  circle A0 centre (-31.5, 68) radius 3
extrude "Extrude1'''''''''''''''''''''''''''''''''''''''''''''''''''" add sketch "Lifter_Pivot_Pin_6mm_Section" along normal blind 72 from surface at -36 separate body makes body 60 in component "Lifter_Pivot_Pin_6mm"
sketch "Servo_30kgcm_Envelope_Only_Outline" plane through (0, 0, 0) normal (0, 0, 1) x (1, 0, 0) in component "Servo_30kgcm_Envelope_Only"
  line L0 (-20, 17) -> (20, 17)
  line L1 (20, 17) -> (20, 57)
  line L2 (20, 57) -> (-20, 57)
  line L3 (-20, 57) -> (-20, 17)
extrude "Extrude1''''''''''''''''''''''''''''''''''''''''''''''''''''" add sketch "Servo_30kgcm_Envelope_Only_Outline" along normal blind 30 from surface at 9 separate body makes body 61 in component "Servo_30kgcm_Envelope_Only"
sketch "Lifter_Servo_Horn_Envelope_Only_Outline" plane through (0, 0, 0) normal (0, 0, 1) x (1, 0, 0) in component "Lifter_Servo_Horn_Envelope_Only"
  line L0 (-4, 48) -> (4, 48)
  line L1 (4, 48) -> (4, 63)
  line L2 (4, 63) -> (-4, 63)
  line L3 (-4, 63) -> (-4, 48)
extrude "Extrude1'''''''''''''''''''''''''''''''''''''''''''''''''''''" add sketch "Lifter_Servo_Horn_Envelope_Only_Outline" along normal blind 3 from surface at 37 separate body makes body 62 in component "Lifter_Servo_Horn_Envelope_Only"
sketch "Lifter_Linkage_Envelope_Only_Outline" plane through (0, 0, 0) normal (0, 0, 1) x (1, 0, 0) in component "Lifter_Linkage_Envelope_Only"
  line L0 (-3, 61) -> (3, 61)
  line L1 (3, 61) -> (3, 72)
  line L2 (3, 72) -> (-3, 72)
  line L3 (-3, 72) -> (-3, 61)
extrude "Extrude1''''''''''''''''''''''''''''''''''''''''''''''''''''''" add sketch "Lifter_Linkage_Envelope_Only_Outline" along normal blind 4 from surface at 34 separate body makes body 63 in component "Lifter_Linkage_Envelope_Only"
sketch "Grabber_Upper_Jaw_Outline" plane through (0, 0, 0) normal (0, 0, 1) x (1, 0, 0) in component "Grabber_Upper_Jaw"
  line L0 (-30, 101) -> (30, 101)
  line L1 (30, 101) -> (30, 109)
  line L2 (30, 109) -> (-30, 109)
  line L3 (-30, 109) -> (-30, 101)
extrude "Extrude1'''''''''''''''''''''''''''''''''''''''''''''''''''''''" add sketch "Grabber_Upper_Jaw_Outline" along normal blind 5 from surface at 44 separate body makes body 64 in component "Grabber_Upper_Jaw"
sketch "Grabber_Arm_L_Outline" plane through (0, 0, 0) normal (0, 0, 1) x (1, 0, 0) in component "Grabber_Arm_L"
  line L0 (-30, 68) -> (-26, 68)
  line L1 (-26, 68) -> (-26, 105)
  line L2 (-26, 105) -> (-30, 105)
  line L3 (-30, 105) -> (-30, 68)
extrude "Extrude1''''''''''''''''''''''''''''''''''''''''''''''''''''''''" add sketch "Grabber_Arm_L_Outline" along normal blind 6 from surface at 45 separate body makes body 65 in component "Grabber_Arm_L"
sketch "Grabber_Arm_R_Outline" plane through (0, 0, 0) normal (0, 0, 1) x (1, 0, 0) in component "Grabber_Arm_R"
  line L0 (26, 68) -> (30, 68)
  line L1 (30, 68) -> (30, 105)
  line L2 (30, 105) -> (26, 105)
  line L3 (26, 105) -> (26, 68)
extrude "Extrude1'''''''''''''''''''''''''''''''''''''''''''''''''''''''''" add sketch "Grabber_Arm_R_Outline" along normal blind 6 from surface at 45 separate body makes body 66 in component "Grabber_Arm_R"
sketch "Sketch1" plane through (0, 0, 0) normal (1, 0, 0) x (0, 0, -1) in component "Grabber_Pivot_Pin_6mm"
  circle A0 centre (-49, 68) radius 3
extrude "Extrude1''''''''''''''''''''''''''''''''''''''''''''''''''''''''''" add sketch "Sketch1" along normal blind 70 from surface at -35 separate body makes body 67 in component "Grabber_Pivot_Pin_6mm"
sketch "Grabber_Pivot_Bracket_L_Outline" plane through (0, 0, 0) normal (0, 0, 1) x (1, 0, 0) in component "Grabber_Pivot_Bracket_L"
  line L0 (-35, 61) -> (-32, 61)
  line L1 (-32, 61) -> (-32, 75)
  line L2 (-32, 75) -> (-35, 75)
  line L3 (-35, 75) -> (-35, 61)
extrude "Extrude1'''''''''''''''''''''''''''''''''''''''''''''''''''''''''''" add sketch "Grabber_Pivot_Bracket_L_Outline" along normal blind 14 from surface at 43 separate body makes body 68 in component "Grabber_Pivot_Bracket_L"
sketch "Grabber_Pivot_Bracket_R_Outline" plane through (0, 0, 0) normal (0, 0, 1) x (1, 0, 0) in component "Grabber_Pivot_Bracket_R"
  line L0 (32, 61) -> (35, 61)
  line L1 (35, 61) -> (35, 75)
  line L2 (35, 75) -> (32, 75)
  line L3 (32, 75) -> (32, 61)
extrude "Extrude1''''''''''''''''''''''''''''''''''''''''''''''''''''''''''''" add sketch "Grabber_Pivot_Bracket_R_Outline" along normal blind 14 from surface at 43 separate body makes body 69 in component "Grabber_Pivot_Bracket_R"
sketch "Grabber_Second_Servo_Envelope_Only_Outline" plane through (0, 0, 0) normal (0, 0, 1) x (1, 0, 0) in component "Grabber_Second_Servo_Envelope_Only"
  line L0 (-15, 23) -> (15, 23)
  line L1 (15, 23) -> (15, 56)
  line L2 (15, 56) -> (-15, 56)
  line L3 (-15, 56) -> (-15, 23)
extrude "Extrude1'''''''''''''''''''''''''''''''''''''''''''''''''''''''''''''" add sketch "Grabber_Second_Servo_Envelope_Only_Outline" along normal blind 26 from surface at 44 separate body makes body 70 in component "Grabber_Second_Servo_Envelope_Only"
sketch "Grabber_Linkage_Envelope_Only_Outline" plane through (0, 0, 0) normal (0, 0, 1) x (1, 0, 0) in component "Grabber_Linkage_Envelope_Only"
  line L0 (-3, 56) -> (3, 56)
  line L1 (3, 56) -> (3, 69)
  line L2 (3, 69) -> (-3, 69)
  line L3 (-3, 69) -> (-3, 56)
extrude "Extrude1''''''''''''''''''''''''''''''''''''''''''''''''''''''''''''''" add sketch "Grabber_Linkage_Envelope_Only_Outline" along normal blind 6 from surface at 53 separate body makes body 71 in component "Grabber_Linkage_Envelope_Only"
sketch "Grabber_Arm_L_6p4mm_Pivot_Clearance" plane through (0, 0, 0) normal (1, 0, 0) x (0, 0, -1) in component "Grabber_Arm_L"
  circle A0 centre (-49, 68) radius 3.2
extrude "Extrude2'''''''''''''''''''''''''''''''''''''''''" cut sketch "Grabber_Arm_L_6p4mm_Pivot_Clearance" along normal mid plane 100 bodies 65 in component "Grabber_Arm_L"
sketch "Grabber_Arm_R_6p4mm_Pivot_Clearance" plane through (0, 0, 0) normal (1, 0, 0) x (0, 0, -1) in component "Grabber_Arm_R"
  circle A0 centre (-49, 68) radius 3.2
extrude "Extrude2''''''''''''''''''''''''''''''''''''''''''" cut sketch "Grabber_Arm_R_6p4mm_Pivot_Clearance" along normal mid plane 100 bodies 66 in component "Grabber_Arm_R"
sketch "Grabber_Pivot_Bracket_L_6p4mm_Pivot_Clearance" plane through (0, 0, 0) normal (1, 0, 0) x (0, 0, -1) in component "Grabber_Pivot_Bracket_L"
  circle A0 centre (-49, 68) radius 3.2
extrude "Extrude2'''''''''''''''''''''''''''''''''''''''''''" cut sketch "Grabber_Pivot_Bracket_L_6p4mm_Pivot_Clearance" along normal mid plane 100 bodies 68 in component "Grabber_Pivot_Bracket_L"
sketch "Grabber_Pivot_Bracket_R_6p4mm_Pivot_Clearance" plane through (0, 0, 0) normal (1, 0, 0) x (0, 0, -1) in component "Grabber_Pivot_Bracket_R"
  circle A0 centre (-49, 68) radius 3.2
extrude "Extrude2''''''''''''''''''''''''''''''''''''''''''''" cut sketch "Grabber_Pivot_Bracket_R_6p4mm_Pivot_Clearance" along normal mid plane 100 bodies 69 in component "Grabber_Pivot_Bracket_R"
sketch "Pin_End_Trim_L" plane through (0, 0, 0) normal (1, 0, 0) x (0, 0, -1) in component "Lifter_Pivot_Pin_6mm"
  circle A0 centre (-31.5, 68) radius 3.5
extrude "Extrude2'''''''''''''''''''''''''''''''''''''''''''''" cut sketch "Pin_End_Trim_L" along normal blind 1.3 from surface at -36.1 bodies 60 in component "Lifter_Pivot_Pin_6mm"
sketch "Pin_End_Trim_R" plane through (0, 0, 0) normal (1, 0, 0) x (0, 0, -1) in component "Lifter_Pivot_Pin_6mm"
  circle A0 centre (-31.5, 68) radius 3.5
extrude "Extrude3''''''''''''''''''''''''" cut sketch "Pin_End_Trim_R" along normal blind 1.3 from surface at 34.8 bodies 60 in component "Lifter_Pivot_Pin_6mm"
sketch "Load_Path_To_Base_L" plane through (0, 0, 0) normal (0, 0, 1) x (1, 0, 0) in component "Lifter_Pivot_Support_L"
  line L0 (-35, 61) -> (-25, 61)
  line L1 (-25, 61) -> (-25, 76)
  line L2 (-25, 76) -> (-35, 76)
  line L3 (-35, 76) -> (-35, 61)
extrude "Extrude3'''''''''''''''''''''''''" add sketch "Load_Path_To_Base_L" along normal blind 20 from surface at 5 bodies 58 in component "Lifter_Pivot_Support_L"
sketch "Lifter_Support_Base_M3_Clear_L" plane through (0, 0, 0) normal (0, 0, 1) x (1, 0, 0) in component "Base_Plate_Al"
  circle A0 centre (-29.5, 64.5) radius 1.7
  circle A1 centre (-29.5, 72.5) radius 1.7
extrude "Lifter_Support_Base_M3_Clear_L_Cut" cut sketch "Lifter_Support_Base_M3_Clear_L" along normal blind 2.2 from surface at 2.9 bodies 1 in component "Base_Plate_Al"
sketch "Lifter_Support_M3_Tap_L" plane through (0, 0, 0) normal (0, 0, 1) x (1, 0, 0) in component "Lifter_Pivot_Support_L"
  circle A0 centre (-29.5, 64.5) radius 1.25
  circle A1 centre (-29.5, 72.5) radius 1.25
extrude "Lifter_Support_M3_Tap_L_Cut" cut sketch "Lifter_Support_M3_Tap_L" along normal blind 8.1 from surface at 4.9 bodies 58 in component "Lifter_Pivot_Support_L"
sketch "Load_Path_To_Base_R" plane through (0, 0, 0) normal (0, 0, 1) x (1, 0, 0) in component "Lifter_Pivot_Support_R"
  line L0 (25, 61) -> (35, 61)
  line L1 (35, 61) -> (35, 76)
  line L2 (35, 76) -> (25, 76)
  line L3 (25, 76) -> (25, 61)
extrude "Extrude3''''''''''''''''''''''''''" add sketch "Load_Path_To_Base_R" along normal blind 20 from surface at 5 bodies 59 in component "Lifter_Pivot_Support_R"
sketch "Lifter_Support_Base_M3_Clear_R" plane through (0, 0, 0) normal (0, 0, 1) x (1, 0, 0) in component "Base_Plate_Al"
  circle A0 centre (29.5, 64.5) radius 1.7
  circle A1 centre (29.5, 72.5) radius 1.7
extrude "Lifter_Support_Base_M3_Clear_R_Cut" cut sketch "Lifter_Support_Base_M3_Clear_R" along normal blind 2.2 from surface at 2.9 bodies 1 in component "Base_Plate_Al"
sketch "Lifter_Support_M3_Tap_R" plane through (0, 0, 0) normal (0, 0, 1) x (1, 0, 0) in component "Lifter_Pivot_Support_R"
  circle A0 centre (29.5, 64.5) radius 1.25
  circle A1 centre (29.5, 72.5) radius 1.25
extrude "Lifter_Support_M3_Tap_R_Cut" cut sketch "Lifter_Support_M3_Tap_R" along normal blind 8.1 from surface at 4.9 bodies 59 in component "Lifter_Pivot_Support_R"
sketch "Repeat_40kg_Servo_MaxEnvelope_Outline" plane through (0, 0, 0) normal (0, 0, 1) x (1, 0, 0) in component "Repeat_40kg_Servo_MaxEnvelope"
  line L0 (-25.1, 12) -> (31.1, 12)
  line L1 (31.1, 12) -> (31.1, 56.5)
  line L2 (31.1, 56.5) -> (-25.1, 56.5)
  line L3 (-25.1, 56.5) -> (-25.1, 12)
extrude "Extrude1'''''''''''''''''''''''''''''''''''''''''''''''''''''''''''''''" add sketch "Repeat_40kg_Servo_MaxEnvelope_Outline" along normal blind 20 from surface at 12 separate body makes body 72 in component "Repeat_40kg_Servo_MaxEnvelope"
sketch "Lifter_Servo_Base_Rail_L_Outline" plane through (0, 0, 0) normal (0, 0, 1) x (1, 0, 0) in component "Lifter_Servo_Base_Rail_L"
  line L0 (-25.1, 14) -> (-21.1, 14)
  line L1 (-21.1, 14) -> (-21.1, 54)
  line L2 (-21.1, 54) -> (-25.1, 54)
  line L3 (-25.1, 54) -> (-25.1, 14)
extrude "Extrude1''''''''''''''''''''''''''''''''''''''''''''''''''''''''''''''''" add sketch "Lifter_Servo_Base_Rail_L_Outline" along normal blind 7 from surface at 5 separate body makes body 73 in component "Lifter_Servo_Base_Rail_L"
sketch "Lifter_Servo_Base_Rail_R_Outline" plane through (0, 0, 0) normal (0, 0, 1) x (1, 0, 0) in component "Lifter_Servo_Base_Rail_R"
  line L0 (27.1, 14) -> (31.1, 14)
  line L1 (31.1, 14) -> (31.1, 54)
  line L2 (31.1, 54) -> (27.1, 54)
  line L3 (27.1, 54) -> (27.1, 14)
extrude "Extrude1'''''''''''''''''''''''''''''''''''''''''''''''''''''''''''''''''" add sketch "Lifter_Servo_Base_Rail_R_Outline" along normal blind 7 from surface at 5 separate body makes body 74 in component "Lifter_Servo_Base_Rail_R"
sketch "Lifter_Aluminium_Horn_Profile" plane through (0, 0, 0) normal (1, 0, 0) x (0, 0, -1) in component "Lifter_Aluminium_Horn"
  line L0 (-25, 38) -> (-25, 61)
  line L1 (-25, 61) -> (-19, 61)
  line L2 (-19, 61) -> (-19, 38)
  line L3 (-19, 38) -> (-25, 38)
extrude "Extrude1''''''''''''''''''''''''''''''''''''''''''''''''''''''''''''''''''" add sketch "Lifter_Aluminium_Horn_Profile" along normal blind 3 from surface at -28.1 separate body makes body 75 in component "Lifter_Aluminium_Horn"
sketch "Lifter_Aluminium_Horn" plane through (0, 0, 0) normal (1, 0, 0) x (0, 0, -1) in component "Lifter_Aluminium_Horn"
  circle A0 centre (-22, 42) radius 1.6
  circle A1 centre (-22, 57) radius 1.6
extrude "Extrude2''''''''''''''''''''''''''''''''''''''''''''''" cut sketch "Lifter_Aluminium_Horn" along normal mid plane 100 bodies 75 in component "Lifter_Aluminium_Horn"
sketch "Lifter_Connecting_Rod_Profile" plane through (0, 0, 0) normal (1, 0, 0) x (0, 0, -1) in component "Lifter_Connecting_Rod"
  line L0 (-18.8868, 53.0875) -> (-49.6277, 61.1068)
  line L1 (-49.6277, 61.1068) -> (-48.1132, 66.9125)
  line L2 (-48.1132, 66.9125) -> (-17.3723, 58.8932)
  line L3 (-17.3723, 58.8932) -> (-18.8868, 53.0875)
extrude "Extrude1'''''''''''''''''''''''''''''''''''''''''''''''''''''''''''''''''''" add sketch "Lifter_Connecting_Rod_Profile" along normal blind 3 from surface at -31.1 separate body makes body 76 in component "Lifter_Connecting_Rod"
sketch "Lifter_Connecting_Rod" plane through (0, 0, 0) normal (1, 0, 0) x (0, 0, -1) in component "Lifter_Connecting_Rod"
  circle A0 centre (-22, 57) radius 1.6
  circle A1 centre (-45, 63) radius 1.6
extrude "Extrude2'''''''''''''''''''''''''''''''''''''''''''''''" cut sketch "Lifter_Connecting_Rod" along normal mid plane 100 bodies 76 in component "Lifter_Connecting_Rod"
sketch "Welded_Lifter_Lever" plane through (0, 0, 0) normal (0, 0, 1) x (1, 0, 0) in component "Lifter_Hinge_Boss"
  line L0 (-28.1, 59) -> (-25.1, 59)
  line L1 (-25.1, 59) -> (-25.1, 69)
  line L2 (-25.1, 69) -> (-28.1, 69)
  line L3 (-28.1, 69) -> (-28.1, 59)
extrude "Extrude3'''''''''''''''''''''''''''" add sketch "Welded_Lifter_Lever" along normal blind 18 from surface at 31 bodies 57 in component "Lifter_Hinge_Boss"
sketch "Lever_M3_Clevis_Hole" plane through (0, 0, 0) normal (1, 0, 0) x (0, 0, -1) in component "Lifter_Hinge_Boss"
  circle A0 centre (-45, 63) radius 1.6
extrude "Extrude4'''''''''''''''''''" cut sketch "Lever_M3_Clevis_Hole" along normal mid plane 100 bodies 57 in component "Lifter_Hinge_Boss"
sketch "Lifter_Lower_Hard_Stop_Outline" plane through (0, 0, 0) normal (0, 0, 1) x (1, 0, 0) in component "Lifter_Lower_Hard_Stop"
  line L0 (-10, 82) -> (10, 82)
  line L1 (10, 82) -> (10, 89)
  line L2 (10, 89) -> (-10, 89)
  line L3 (-10, 89) -> (-10, 82)
extrude "Extrude1''''''''''''''''''''''''''''''''''''''''''''''''''''''''''''''''''''" add sketch "Lifter_Lower_Hard_Stop_Outline" along normal blind 8 from surface at 5 separate body makes body 77 in component "Lifter_Lower_Hard_Stop"
sketch "Servo_Output_Shaft_D3" plane through (0, 0, 0) normal (1, 0, 0) x (0, 0, -1) in component "Repeat_40kg_Servo_MaxEnvelope"
  circle A0 centre (-22, 42) radius 1.5
extrude "Extrude2''''''''''''''''''''''''''''''''''''''''''''''''" add sketch "Servo_Output_Shaft_D3" along normal blind 4 from surface at -28.1 bodies 72 in component "Repeat_40kg_Servo_MaxEnvelope"
sketch "Flange_Clearance_L" plane through (0, 0, 0) normal (0, 0, 1) x (1, 0, 0) in component "Lifter_Pivot_Support_L"
  line L0 (-32, 60.9) -> (-24.9, 60.9)
  line L1 (-24.9, 60.9) -> (-24.9, 76.1)
  line L2 (-24.9, 76.1) -> (-32, 76.1)
  line L3 (-32, 76.1) -> (-32, 60.9)
extrude "Extrude5'''''''''''" cut sketch "Flange_Clearance_L" along normal blind 11.1 from surface at 14 bodies 58 in component "Lifter_Pivot_Support_L"
sketch "Flange_Clearance_R" plane through (0, 0, 0) normal (0, 0, 1) x (1, 0, 0) in component "Lifter_Pivot_Support_R"
  line L0 (24.9, 60.9) -> (32, 60.9)
  line L1 (32, 60.9) -> (32, 76.1)
  line L2 (32, 76.1) -> (24.9, 76.1)
  line L3 (24.9, 76.1) -> (24.9, 60.9)
extrude "Extrude5''''''''''''" cut sketch "Flange_Clearance_R" along normal blind 11.1 from surface at 14 bodies 59 in component "Lifter_Pivot_Support_R"
sketch "Lever_Repair_Pivot_Bore" plane through (0, 0, 0) normal (1, 0, 0) x (0, 0, -1) in component "Lifter_Hinge_Boss"
  circle A0 centre (-31.5, 68) radius 3.2
extrude "Extrude5'''''''''''''" cut sketch "Lever_Repair_Pivot_Bore" along normal mid plane 100 bodies 57 in component "Lifter_Hinge_Boss"